Autodesk Inventor part; units mm, degrees
(part 2 of 2)
sketch "스케치9" plane through (23.3709, 0, 32.592) normal (0, 0, 1) x (-1, 0, 0)
  line L0 (52.8167, 0) -> (53.5238, 0) projected
  line L1 (53.5238, 0) -> (52.8167, 0) projected
  line L2 (54.2309, 0) -> (53.5238, 0) projected
  line L3 (54.938, 0) -> (54.2309, 0) projected
  line L4 (54.2309, 0) -> (54.938, 0) projected
  line L5 (54.938, 0) -> (54.2309, 0) projected
  line L6 (55.6451, 0) -> (54.938, 0) projected
  line L7 (56.3522, 0) -> (55.6451, 0) projected
  line L8 (55.6451, 0) -> (56.3522, 0) projected
  line L9 (56.3522, 0) -> (55.6451, 0) projected
  line L10 (57.0593, 0) -> (56.3522, 0) projected
  line L11 (57.7664, 0) -> (57.0593, 0) projected
  line L12 (57.0593, 0) -> (57.7664, 0) projected
  line L13 (57.7664, 0) -> (57.0593, 0) projected
  line L14 (58.4735, 0) -> (57.7664, 0) projected
  line L15 (59.1806, 0) -> (58.4735, 0) projected
  line L16 (58.4735, 0) -> (59.1806, 0) projected
  line L17 (59.1806, 0) -> (58.4735, 0) projected
  line L18 (59.8877, 0) -> (59.1806, 0) projected
  line L19 (60.5948, 0) -> (59.8877, 0) projected
  line L20 (59.8877, 0) -> (60.5948, 0) projected
  line L21 (60.5948, 0) -> (59.8877, 0) projected
  line L22 (61.3019, 0) -> (60.5948, 0) projected
  line L23 (62.0091, 0) -> (61.3019, 0) projected
  line L24 (61.3019, 0) -> (62.0091, 0) projected
  line L25 (62.0091, 0) -> (61.3019, 0) projected
  line L26 (62.7162, 0) -> (62.0091, 0) projected
  line L27 (63.4233, 0) -> (62.7162, 0) projected
  line L28 (62.7162, 0) -> (63.4233, 0) projected
  line L29 (63.4233, 0) -> (62.7162, 0) projected
  line L30 (64.1304, 0) -> (63.4233, 0) projected
  line L31 (64.8375, 0) -> (64.1304, 0) projected
  line L32 (64.1304, 0) -> (64.8375, 0) projected
  line L33 (64.8375, 0) -> (64.1304, 0) projected
  line L34 (65.5446, 0) -> (64.8375, 0) projected
  line L35 (66.2517, 0) -> (65.5446, 0) projected
  line L36 (65.5446, 0) -> (66.2517, 0) projected
  line L37 (66.2517, 0) -> (65.5446, 0) projected
  line L38 (66.9588, 0) -> (66.2517, 0) projected
  line L39 (68.539, 0) -> (66.9588, 0) projected
  line L40 (67.539, 0) -> (68.539, 0) projected
  line L41 (68.539, 0) -> (67.539, 0) projected
  line L42 (67.539, 0) -> (68.539, 0) projected
  line L43 (68.539, 0) -> (67.539, 0) projected
  line L44 (67.539, 0) -> (68.539, 0) projected
  line L45 (68.539, 0) -> (67.539, 0) projected
  line L46 (67.539, 0) -> (68.539, 0) projected
  line L47 (68.539, 0) -> (67.539, 0) projected
  line L48 (67.539, 0) -> (68.539, 0) projected
  line L49 (68.539, 0) -> (67.539, 0) projected
  line L50 (67.539, 0) -> (68.539, 0) projected
  line L51 (68.539, 0) -> (67.539, 0) projected
  line L52 (67.539, 0) -> (68.539, 0) projected
  line L53 (68.539, 0) -> (67.539, 0) projected
  line L54 (67.539, 0) -> (68.539, 0) projected
  line L55 (68.539, 0) -> (67.539, 0) projected
  line L56 (67.539, 0) -> (68.539, 0) projected
  line L57 (68.539, 0) -> (67.539, 0) projected
  line L58 (67.539, 0) -> (68.539, 0) projected
  line L59 (68.539, 0) -> (67.539, 0) projected
  line L60 (67.539, 0) -> (68.539, 0) projected
  line L61 (68.539, 0) -> (67.539, 0) projected
  line L62 (67.539, 0) -> (68.539, 0) projected
  line L63 (68.539, 0) -> (67.539, 0) projected
  line L64 (67.8319, 0) -> (68.539, 0) projected
  line L65 (67.1248, 0) -> (67.8319, 0) projected
  line L66 (66.4177, 0) -> (67.1248, 0) projected
  line L67 (67.1248, 0) -> (66.4177, 0) projected
  line L68 (66.4177, 0) -> (67.1248, 0) projected
  line L69 (65.7106, 0) -> (66.4177, 0) projected
  line L70 (65.0035, 0) -> (65.7106, 0) projected
  line L71 (65.7106, 0) -> (65.0035, 0) projected
  line L72 (65.0035, 0) -> (65.7106, 0) projected
  line L73 (64.2964, 0) -> (65.0035, 0) projected
  line L74 (63.5892, 0) -> (64.2964, 0) projected
  line L75 (64.2964, 0) -> (63.5892, 0) projected
  line L76 (63.5892, 0) -> (64.2964, 0) projected
  line L77 (62.8821, 0) -> (63.5892, 0) projected
  line L78 (62.175, 0) -> (62.8821, 0) projected
  line L79 (62.8821, 0) -> (62.175, 0) projected
  line L80 (62.175, 0) -> (62.8821, 0) projected
  line L81 (61.4679, 0) -> (62.175, 0) projected
  line L82 (60.7608, 0) -> (61.4679, 0) projected
  line L83 (61.4679, 0) -> (60.7608, 0) projected
  line L84 (60.7608, 0) -> (61.4679, 0) projected
  line L85 (60.0537, 0) -> (60.7608, 0) projected
  line L86 (59.3466, 0) -> (60.0537, 0) projected
  line L87 (60.0537, 0) -> (59.3466, 0) projected
  line L88 (59.3466, 0) -> (60.0537, 0) projected
  line L89 (58.6395, 0) -> (59.3466, 0) projected
  line L90 (57.9324, 0) -> (58.6395, 0) projected
  line L91 (58.6395, 0) -> (57.9324, 0) projected
  line L92 (57.9324, 0) -> (58.6395, 0) projected
  line L93 (57.2253, 0) -> (57.9324, 0) projected
  line L94 (56.5182, 0) -> (57.2253, 0) projected
  line L95 (57.2253, 0) -> (56.5182, 0) projected
  line L96 (56.5182, 0) -> (57.2253, 0) projected
  line L97 (55.8111, 0) -> (56.5182, 0) projected
  line L98 (55.104, 0) -> (55.8111, 0) projected
  line L99 (55.8111, 0) -> (55.104, 0) projected
  line L100 (55.104, 0) -> (55.8111, 0) projected
  line L101 (54.3969, 0) -> (55.104, 0) projected
  line L102 (53.6898, 0) -> (54.3969, 0) projected
  line L103 (54.3969, 0) -> (53.6898, 0) projected
  line L104 (53.6898, 0) -> (54.3969, 0) projected
  line L105 (52.9826, 0) -> (53.6898, 0) projected
  line L106 (52.2755, 0) -> (52.9826, 0) projected
  line L107 (52.9826, 0) -> (52.2755, 0) projected
  line L108 (52.2755, 0) -> (52.9826, 0) projected
  line L109 (51.5684, 0) -> (52.2755, 0) projected
  line L110 (50.8613, 0) -> (51.5684, 0) projected
  line L111 (51.5684, 0) -> (50.8613, 0) projected
  line L112 (49.9882, 0) -> (51.5684, 0) projected
  line L113 (48.9882, 0) -> (49.9882, 0) projected
  line L114 (47.9882, 0) -> (48.9882, 0) projected
  line L115 (46.9882, 0) -> (47.9882, 0) projected
  line L116 (45.9882, 0) -> (46.9882, 0) projected
  line L117 (44.9882, 0) -> (45.9882, 0) projected
  line L118 (43.9882, 0) -> (44.9882, 0) projected
  line L119 (42.9882, 0) -> (43.9882, 0) projected
  line L120 (41.9882, 0) -> (42.9882, 0) projected
  line L121 (40.9882, 0) -> (41.9882, 0) projected
  line L122 (39.9882, 0) -> (40.9882, 0) projected
  line L123 (38.9882, 0) -> (39.9882, 0) projected
  line L124 (37.9882, 0) -> (38.9882, 0) projected
  line L125 (36.9882, 0) -> (37.9882, 0) projected
  line L126 (35.9882, 0) -> (36.9882, 0) projected
  line L127 (34.9882, 0) -> (35.9882, 0) projected
  line L128 (33.9882, 0) -> (34.9882, 0) projected
  line L129 (32.9882, 0) -> (33.9882, 0) projected
  line L130 (31.9882, 0) -> (32.9882, 0) projected
  line L131 (30.9882, 0) -> (31.9882, 0) projected
  line L132 (29.9882, 0) -> (30.9882, 0) projected
  line L133 (28.9882, 0) -> (29.9882, 0) projected
  line L134 (27.9882, 0) -> (28.9882, 0) projected
  line L135 (26.9882, 0) -> (27.9882, 0) projected
  line L136 (25.9882, 0) -> (26.9882, 0) projected
  line L137 (23.7535, 0) -> (25.9882, 0) projected
  line L138 (23.0464, 0) -> (23.7535, 0) projected
  line L139 (23.7535, 0) -> (23.0464, 0) projected
  line L140 (23.0464, 0) -> (23.7535, 0) projected
  line L141 (22.3393, 0) -> (23.0464, 0) projected
  line L142 (21.6322, 0) -> (22.3393, 0) projected
  line L143 (22.3393, 0) -> (21.6322, 0) projected
  line L144 (21.6322, 0) -> (22.3393, 0) projected
  line L145 (20.9251, 0) -> (21.6322, 0) projected
  line L146 (20.218, 0) -> (20.9251, 0) projected
  line L147 (20.9251, 0) -> (20.218, 0) projected
  line L148 (20.218, 0) -> (20.9251, 0) projected
  line L149 (19.5109, 0) -> (20.218, 0) projected
  line L150 (18.8038, 0) -> (19.5109, 0) projected
  line L151 (19.5109, 0) -> (18.8038, 0) projected
  line L152 (18.8038, 0) -> (19.5109, 0) projected
  line L153 (18.0967, 0) -> (18.8038, 0) projected
  line L154 (17.3895, 0) -> (18.0967, 0) projected
  line L155 (18.0967, 0) -> (17.3895, 0) projected
  line L156 (17.3895, 0) -> (18.0967, 0) projected
  line L157 (16.6824, 0) -> (17.3895, 0) projected
  line L158 (15.9753, 0) -> (16.6824, 0) projected
  line L159 (16.6824, 0) -> (15.9753, 0) projected
  line L160 (15.9753, 0) -> (16.6824, 0) projected
  line L161 (15.2682, 0) -> (15.9753, 0) projected
  line L162 (14.5611, 0) -> (15.2682, 0) projected
  line L163 (15.2682, 0) -> (14.5611, 0) projected
  line L164 (14.5611, 0) -> (15.2682, 0) projected
  line L165 (13.854, 0) -> (14.5611, 0) projected
  line L166 (13.1469, 0) -> (13.854, 0) projected
  line L167 (13.854, 0) -> (13.1469, 0) projected
  line L168 (13.1469, 0) -> (13.854, 0) projected
  line L169 (12.4398, 0) -> (13.1469, 0) projected
  line L170 (11.7327, 0) -> (12.4398, 0) projected
  line L171 (12.4398, 0) -> (11.7327, 0) projected
  line L172 (11.7327, 0) -> (12.4398, 0) projected
  line L173 (11.0256, 0) -> (11.7327, 0) projected
  line L174 (10.3185, 0) -> (11.0256, 0) projected
  line L175 (11.0256, 0) -> (10.3185, 0) projected
  line L176 (10.3185, 0) -> (11.0256, 0) projected
  line L177 (9.6114, 0) -> (10.3185, 0) projected
  line L178 (8.9043, 0) -> (9.6114, 0) projected
  line L179 (9.6114, 0) -> (8.9043, 0) projected
  line L180 (8.9043, 0) -> (9.6114, 0) projected
  line L181 (8.1972, 0) -> (8.9043, 0) projected
  line L182 (7.4901, 0) -> (8.1972, 0) projected
  line L183 (8.1972, 0) -> (7.4901, 0) projected
  line L184 (7.4901, 0) -> (8.1972, 0) projected
  line L185 (6.7829, 0) -> (7.4901, 0) projected
  line L186 (5.2028, 0) -> (6.7829, 0) projected
  line L187 (6.2028, 0) -> (5.2028, 0) projected
  line L188 (5.2028, 0) -> (6.2028, 0) projected
  line L189 (6.2028, 0) -> (5.2028, 0) projected
  line L190 (5.2028, 0) -> (6.2028, 0) projected
  line L191 (6.2028, 0) -> (5.2028, 0) projected
  line L192 (5.2028, 0) -> (6.2028, 0) projected
  line L193 (6.2028, 0) -> (5.2028, 0) projected
  line L194 (5.2028, 0) -> (6.2028, 0) projected
  line L195 (6.2028, 0) -> (5.2028, 0) projected
  line L196 (5.2028, 0) -> (6.2028, 0) projected
  line L197 (6.2028, 0) -> (5.2028, 0) projected
  line L198 (5.2028, 0) -> (6.2028, 0) projected
  line L199 (6.2028, 0) -> (5.2028, 0) projected
  line L200 (5.2028, 0) -> (6.2028, 0) projected
  line L201 (6.2028, 0) -> (5.2028, 0) projected
  line L202 (5.2028, 0) -> (6.2028, 0) projected
  line L203 (6.2028, 0) -> (5.2028, 0) projected
  line L204 (5.2028, 0) -> (6.2028, 0) projected
  line L205 (6.2028, 0) -> (5.2028, 0) projected
  line L206 (5.2028, 0) -> (6.2028, 0) projected
  line L207 (6.2028, 0) -> (5.2028, 0) projected
  line L208 (5.2028, 0) -> (6.2028, 0) projected
  line L209 (6.2028, 0) -> (5.2028, 0) projected
  line L210 (5.2028, 0) -> (6.2028, 0) projected
  line L211 (5.9099, 0) -> (5.2028, 0) projected
  line L212 (6.617, 0) -> (5.9099, 0) projected
  line L213 (7.3241, 0) -> (6.617, 0) projected
  line L214 (6.617, 0) -> (7.3241, 0) projected
  line L215 (7.3241, 0) -> (6.617, 0) projected
  line L216 (8.0312, 0) -> (7.3241, 0) projected
  line L217 (8.7383, 0) -> (8.0312, 0) projected
  line L218 (8.0312, 0) -> (8.7383, 0) projected
  line L219 (8.7383, 0) -> (8.0312, 0) projected
  line L220 (9.4454, 0) -> (8.7383, 0) projected
  line L221 (10.1525, 0) -> (9.4454, 0) projected
  line L222 (9.4454, 0) -> (10.1525, 0) projected
  line L223 (10.1525, 0) -> (9.4454, 0) projected
  line L224 (10.8596, 0) -> (10.1525, 0) projected
  line L225 (11.5667, 0) -> (10.8596, 0) projected
  line L226 (10.8596, 0) -> (11.5667, 0) projected
  line L227 (11.5667, 0) -> (10.8596, 0) projected
  line L228 (12.2738, 0) -> (11.5667, 0) projected
  line L229 (12.9809, 0) -> (12.2738, 0) projected
  line L230 (12.2738, 0) -> (12.9809, 0) projected
  line L231 (12.9809, 0) -> (12.2738, 0) projected
  line L232 (13.688, 0) -> (12.9809, 0) projected
  line L233 (14.3951, 0) -> (13.688, 0) projected
  line L234 (13.688, 0) -> (14.3951, 0) projected
  line L235 (14.3951, 0) -> (13.688, 0) projected
  line L236 (15.1022, 0) -> (14.3951, 0) projected
  line L237 (15.8094, 0) -> (15.1022, 0) projected
  line L238 (15.1022, 0) -> (15.8094, 0) projected
  line L239 (15.8094, 0) -> (15.1022, 0) projected
  line L240 (16.5165, 0) -> (15.8094, 0) projected
  line L241 (17.2236, 0) -> (16.5165, 0) projected
  line L242 (16.5165, 0) -> (17.2236, 0) projected
  line L243 (17.2236, 0) -> (16.5165, 0) projected
  line L244 (17.9307, 0) -> (17.2236, 0) projected
  line L245 (18.6378, 0) -> (17.9307, 0) projected
  line L246 (17.9307, 0) -> (18.6378, 0) projected
  line L247 (18.6378, 0) -> (17.9307, 0) projected
  line L248 (19.3449, 0) -> (18.6378, 0) projected
  line L249 (20.052, 0) -> (19.3449, 0) projected
  line L250 (19.3449, 0) -> (20.052, 0) projected
  line L251 (20.052, 0) -> (19.3449, 0) projected
  line L252 (20.7591, 0) -> (20.052, 0) projected
  line L253 (21.4662, 0) -> (20.7591, 0) projected
  line L254 (20.7591, 0) -> (21.4662, 0) projected
  line L255 (21.4662, 0) -> (20.7591, 0) projected
  line L256 (22.1733, 0) -> (21.4662, 0) projected
  line L257 (22.8804, 0) -> (22.1733, 0) projected
  line L258 (22.1733, 0) -> (22.8804, 0) projected
  line L259 (23.7535, 0) -> (22.1733, 0) projected
  line L260 (24.7535, 0) -> (23.7535, 0) projected
  line L261 (25.7535, 0) -> (24.7535, 0) projected
  line L262 (26.7535, 0) -> (25.7535, 0) projected
  line L263 (27.7535, 0) -> (26.7535, 0) projected
  line L264 (28.7535, 0) -> (27.7535, 0) projected
  line L265 (29.7535, 0) -> (28.7535, 0) projected
  line L266 (30.7535, 0) -> (29.7535, 0) projected
  line L267 (31.7535, 0) -> (30.7535, 0) projected
  line L268 (32.7535, 0) -> (31.7535, 0) projected
  line L269 (33.7535, 0) -> (32.7535, 0) projected
  line L270 (34.7535, 0) -> (33.7535, 0) projected
  line L271 (35.7535, 0) -> (34.7535, 0) projected
  line L272 (36.7535, 0) -> (35.7535, 0) projected
  line L273 (37.7535, 0) -> (36.7535, 0) projected
  line L274 (38.7535, 0) -> (37.7535, 0) projected
  line L275 (39.7535, 0) -> (38.7535, 0) projected
  line L276 (40.7535, 0) -> (39.7535, 0) projected
  line L277 (41.7535, 0) -> (40.7535, 0) projected
  line L278 (42.7535, 0) -> (41.7535, 0) projected
  line L279 (43.7535, 0) -> (42.7535, 0) projected
  line L280 (44.7535, 0) -> (43.7535, 0) projected
  line L281 (45.7535, 0) -> (44.7535, 0) projected
  line L282 (46.7535, 0) -> (45.7535, 0) projected
  line L283 (47.7535, 0) -> (46.7535, 0) projected
  line L284 (49.9882, 0) -> (47.7535, 0) projected
  line L285 (50.6953, 0) -> (49.9882, 0) projected
  line L286 (49.9882, 0) -> (50.6953, 0) projected
  line L287 (50.6953, 0) -> (49.9882, 0) projected
  line L288 (51.4025, 0) -> (50.6953, 0) projected
  line L289 (52.1096, 0) -> (51.4025, 0) projected
  line L290 (51.4025, 0) -> (52.1096, 0) projected
  line L291 (52.1096, 0) -> (51.4025, 0) projected
  line L292 (52.8167, 0) -> (52.1096, 0) projected
  line L293 (53.5238, 0) -> (52.8167, 0) projected
  line L294 (55.8111, 0) -> (45.8111, 0)
  line L295 (46.9882, 10) -> (46.9882, 0)
  line L296 (46.9882, 0) -> (56.9882, 0)
  line L297 (56.9882, 0) -> (56.9882, 10)
  line L298 (36.8708, 0) -> (36.8708, 30.3476)
  arc A0 (56.9882, 10) -> (46.9882, 10) centre (51.9882, 10) ccw
  circle A1 centre (51.9882, 10) radius 1.25
  line L299 (26.7533, 10) -> (26.7533, 0)
  line L300 (16.7533, 0) -> (16.7533, 10)
  arc A2 (26.7533, 10) -> (16.7533, 10) centre (21.7533, 10) ccw
  circle A3 centre (21.7533, 10) radius 1.25
  point P0 (23.3709, 0)
  point P1 (36.8708, 0)
  point P2 (56.1646, 0)
  point P3 (16.7533, 0)
  point P4 (17.3895, 0)
  point P5 (48.9882, 0)
  point P6 (50.8613, 0)
  point P7 (52.2755, 0)
  point P8 (52.8167, 0)
  point P9 (56.9882, 0)
  dimension "d39" = 0
  dimension "d40" = 2.5
  constraints: 14 end point, 6 symmetric about line, 4 centre point, 4 point on circle, 3 coincident, 1 horizontal, 1 midpoint, 1 parallel, 1 vertical, 2 other
  measures "d39" distance from line of point (56.165, 0) L296
  measures "d40" diameter of A1
extrude "돌출5" add sketch "스케치9" along normal mid plane 5
sketch "스케치10" plane through (0, 0, 0) normal (0, -1, 0) x (1, 0, 0)
  circle A0 centre (-13.5722, 14.7206) radius 1.25
  point P0 (0, 0)
  dimension "d43" = 2.5
  constraints: 1 centre point
  measures "d43" diameter of A0
extrude "돌출6" cut sketch "스케치10" against normal blind 5
